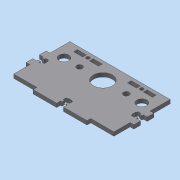
# Autodesk Inventor part: X-Anchor_Front-Outer
Saved by Autodesk Inventor 2016 SP1 (Build 200210100, 210)
## iProperties
Created: 2015-12-01
Part Number: X-Anchor_Front-Outer
Material: Generic
Document SubType Name: Modeling
Designer: Mohamed A.
Density: 1 g/cm^3
Appearance: Default
Author: Mohamed A.
Autodesk Inventor part; units mm, degrees
ref_plane "YZ Plane" through (0, 0, 0) normal (1, 0, 0) x (0, 1, 0)
ref_plane "XZ Plane" through (0, 0, 0) normal (0, 1, 0) x (-1, 0, 0)
ref_plane "XY Plane" through (0, 0, 0) normal (0, 0, 1) x (1, 0, 0)
sketch "Sketch1" plane through (0, 0, 0) normal (0, 0, 1) x (1, 0, 0)
  circle A0 centre (0, 5) radius 7.5
  line L0 (42.7333, 18.5) -> (-42.7333, 18.5)
  line L1 (-42.7333, -29) -> (42.7333, -29)
  circle A1 centre (18.5, 5) radius 2.25
  circle A2 centre (-18.5, 5) radius 2.25
  circle A3 centre (30.8333, 5) radius 3.9
  circle A4 centre (-30.8333, 5) radius 3.9
  line L2 (42.7333, 18.5) -> (42.7333, -29)
  line L3 (-42.7333, -29) -> (-42.7333, 18.5)
  circle A5 centre (0, 5) radius 13.5 construction
  line L4 (0, 41.7106) -> (0, -39.2634) construction
  dimension "d2" = 4.5
  dimension "d3" = 4.5
  dimension "d4" = 7.8
  dimension "d5" = 7.8
  dimension "d48" = 47.5
  dimension "d58" = 15
  dimension "d63" = 27
  dimension "d75" = 34
  dimension "d76" = 30.8333
  dimension "d77" = 85.4667
  dimension "d93" = 47.5
  dimension "d99" = 61.667
  constraints: 10 end point, 6 centre point, 3 vertical, 1 coincident, 1 perpendicular, 1 point on line, 6 other
  measures "d2" diameter of A1
  measures "d3" diameter of A2
  measures "d4" diameter of A3
  measures "d5" diameter of A4
  measures "d48" distance between parallel lines of L1 L0
  measures "d58" diameter of A0
  measures "d63" diameter of A5
  measures "d75" distance from line of A0.centre L1
  measures "d76" distance from line of A3.centre L4
  measures "d77" distance between parallel lines of L3 L2
  measures "d93" distance of L0.start L1.end
extrude "Extrusion1" add sketch "Sketch1" against normal blind 3
sketch "Sketch4" plane through (0, 0, 0) normal (0, 0, 1) x (1, 0, 0)
  line L0 (42.7333, 18.5) -> (39.7333, 18.5)
  line L1 (-42.7333, 18.5) -> (-39.7333, 18.5)
  line L2 (42.7333, -29) -> (21.3667, -29)
  line L3 (21.3667, -26) -> (39.7333, -26)
  line L4 (-42.7333, -29) -> (-21.3667, -29)
  line L5 (-21.3667, -29) -> (-21.3667, -26)
  line L6 (-21.3667, -26) -> (-39.7333, -26)
  line L7 (-42.7333, -23) -> (-42.7333, -29)
  line L8 (42.7333, 18.5) -> (39.7333, 18.5)
  line L9 (39.7333, 18.5) -> (39.7333, 2.6667)
  line L10 (39.7333, 2.6667) -> (42.7333, 2.6667)
  line L11 (42.7333, 2.6667) -> (42.7333, 18.5)
  line L12 (39.7333, -26) -> (39.7333, -13.1667)
  line L13 (39.7333, -13.1667) -> (42.7333, -13.1667)
  line L14 (-42.7333, 2.6667) -> (-39.7333, 2.6667)
  line L15 (-39.7333, 2.6667) -> (-39.7333, 18.5)
  line L16 (-39.7333, 18.5) -> (-42.7333, 18.5)
  line L17 (-42.7333, 18.5) -> (-42.7333, 2.6667)
  line L18 (-42.7333, -29) -> (-39.7333, -29)
  line L19 (-39.7333, -26) -> (-39.7333, -13.1667)
  line L20 (-39.7333, -13.1667) -> (-42.7333, -13.1667)
  line L21 (-42.7333, -13.1667) -> (-42.7333, -29)
  line L22 (21.3667, -29) -> (21.3667, -26)
  line L23 (-21.3667, -23) -> (-21.3667, -29)
  line L24 (-42.7333, 18.5) -> (-39.7333, 18.5)
  line L25 (-42.7333, -29) -> (42.7333, -29) projected
  line L26 (42.7333, 18.5) -> (-42.7333, 18.5) projected
  line L27 (50.1623, -5.25) -> (-50.4474, -5.25) construction
  line L28 (42.7333, -29) -> (42.7333, 18.5) projected
  line L29 (42.7333, -3.75) -> (34.7333, -3.75)
  line L30 (34.7333, -3.75) -> (34.7333, -6.75)
  line L31 (34.7333, -6.75) -> (42.7333, -6.75)
  line L32 (42.7333, -6.75) -> (42.7333, -3.75)
  circle A0 centre (0, 5) radius 13.5 construction
  circle A1 centre (0, 5) radius 7.5
  line L33 (42.7333, -2.6) -> (39.7333, -2.6)
  line L34 (39.7333, -2.6) -> (39.7333, -7.9)
  line L35 (39.7333, -7.9) -> (42.7333, -7.9)
  line L36 (42.7333, -7.9) -> (42.7333, -2.6)
  line L37 (35.3333, -2.6) -> (37.7333, -2.6)
  line L38 (37.7333, -2.6) -> (37.7333, -7.9)
  line L39 (37.7333, -7.9) -> (35.3333, -7.9)
  line L40 (35.3333, -7.9) -> (35.3333, -2.6)
  line L41 (0, 33.7344) -> (0, -36.9537) construction
  line L42 (-42.7333, 18.5) -> (-42.7333, -29) projected
  line L43 (-42.7333, -3.75) -> (-34.7333, -3.75)
  line L44 (-34.7333, -3.75) -> (-34.7333, -6.75)
  line L45 (-34.7333, -6.75) -> (-42.7333, -6.75)
  line L46 (-42.7333, -6.75) -> (-42.7333, -3.75)
  line L47 (-42.7333, -2.6) -> (-39.7333, -2.6)
  line L48 (-39.7333, -2.6) -> (-39.7333, -7.9)
  line L49 (-39.7333, -7.9) -> (-42.7333, -7.9)
  line L50 (-42.7333, -7.9) -> (-42.7333, -2.6)
  line L51 (-35.3333, -2.6) -> (-37.7333, -2.6)
  line L52 (-37.7333, -2.6) -> (-37.7333, -7.9)
  line L53 (-37.7333, -7.9) -> (-35.3333, -7.9)
  line L54 (-35.3333, -7.9) -> (-35.3333, -2.6)
  line L55 (42.7333, -29) -> (-42.7333, -29) projected
  line L56 (-1.5, -29) -> (1.5, -29)
  line L57 (1.5, -29) -> (1.5, -21)
  line L58 (1.5, -21) -> (-1.5, -21)
  line L59 (-1.5, -21) -> (-1.5, -29)
  line L60 (-2.65, -29) -> (2.65, -29)
  line L61 (2.65, -29) -> (2.65, -26)
  line L62 (2.65, -26) -> (-2.65, -26)
  line L63 (-2.65, -26) -> (-2.65, -29)
  line L64 (-2.65, -21.6) -> (2.65, -21.6)
  line L65 (2.65, -21.6) -> (2.65, -24)
  line L66 (2.65, -24) -> (-2.65, -24)
  line L67 (-2.65, -24) -> (-2.65, -21.6)
  line L68 (31.3, 16) -> (24.0167, 16) construction
  line L69 (11.4333, 16) -> (11.4333, 13) construction
  line L70 (11.4333, 13) -> (18.7167, 13) construction
  line L71 (31.3, 13) -> (31.3, 16) construction
  circle A2 centre (30.8333, 5) radius 3.9 projected
  line L72 (21.3667, 17.602) -> (21.3667, 7.8585) construction
  line L73 (18.7167, 16) -> (24.0167, 16) construction
  line L74 (24.0167, 16) -> (24.0167, 13) construction
  line L75 (24.0167, 13) -> (18.7167, 13) construction
  line L76 (18.7167, 13) -> (18.7167, 16) construction
  line L77 (18.7167, 16) -> (11.4333, 16) construction
  line L78 (24.0167, 13) -> (31.3, 13) construction
  circle A3 centre (21.3667, 14.5) radius 1.4
  line L79 (-31.3, 16) -> (-24.0167, 16) construction
  line L80 (-11.4333, 16) -> (-11.4333, 13) construction
  line L81 (-11.4333, 13) -> (-18.7167, 13) construction
  line L82 (-31.3, 13) -> (-31.3, 16) construction
  line L83 (-24.0167, 16) -> (-24.0167, 13) construction
  line L84 (-18.7167, 13) -> (-18.7167, 16) construction
  line L85 (-18.7167, 16) -> (-11.4333, 16) construction
  line L86 (-24.0167, 13) -> (-31.3, 13) construction
  circle A4 centre (-21.3667, 14.5) radius 1.4
  line L87 (42.7333, 18.5) -> (42.7333, -29) projected
  line L88 (42.7333, -13.1667) -> (42.7333, -29)
  line L89 (11.4247, 13) -> (11.4247, 16)
  line L90 (11.4247, 16) -> (18.7077, 16)
  line L91 (18.7077, 16) -> (18.7077, 13)
  line L92 (18.7077, 13) -> (11.4247, 13)
  line L93 (31.2907, 16) -> (31.2907, 13)
  line L94 (31.2907, 13) -> (24.0077, 13)
  line L95 (24.0077, 13) -> (24.0077, 16)
  line L96 (24.0077, 16) -> (31.2907, 16)
  line L97 (-18.7073, 13) -> (-18.7073, 16)
  line L98 (-18.7073, 16) -> (-11.4243, 16)
  line L99 (-11.4243, 16) -> (-11.4243, 13)
  line L100 (-11.4243, 13) -> (-18.7073, 13)
  line L101 (-24.0073, 16) -> (-24.0073, 13)
  line L102 (-24.0073, 13) -> (-31.2903, 13)
  line L103 (-31.2903, 13) -> (-31.2903, 16)
  line L104 (-31.2903, 16) -> (-24.0073, 16)
  dimension "d25" = 3
  dimension "d26" = 3
  dimension "d33" = 15.8333
  dimension "d59" = 8
  dimension "d60" = 3
  dimension "d61" = 47.5
  dimension "d62" = 27
  dimension "d65" = 5.3
  dimension "d66" = 2.4
  dimension "d68" = 5
  dimension "d69" = 3
  dimension "d70" = 8
  dimension "d71" = 5.3
  dimension "d74" = 5
  dimension "d78" = 3
  dimension "d81" = 3
  dimension "d82" = 11
  dimension "d83" = 19.8667
  dimension "d85" = 79.4667
  dimension "d86" = 85.4667
  dimension "d87" = 3
  dimension "d88" = 5.3
  dimension "d89" = 2.8
  dimension "d91" = 15.8333
  dimension "d92" = 21.3667
  dimension "d94" = 2.4
  dimension "d95" = 2.4
  dimension "d96" = 11.4333
  dimension "d97" = 7.2833
  dimension "d98" = 2.65
  constraints: 198 end point, 29 parallel, 25 horizontal, 21 symmetric about line, 15 collinear, 13 perpendicular, 10 point on line, 10 vertical, 4 centre point, 3 equal length, 1 concentric, 27 other
  measures "d25" distance of L2.end L3.start
  measures "d26" distance of L5.end L4.end
  measures "d33" distance from line of L0.start L10
  measures "d59" distance of L31.end L30.end
  measures "d60" distance of L30.end L29.end
  measures "d61" distance between parallel lines of L25 L26
  measures "d62" diameter of A0
  measures "d65" distance of L34.end L33.end
  measures "d66" distance of L38.end L39.end
  measures "d68" distance between parallel lines of L36 L38
  measures "d69" distance of L58.end L57.end
  measures "d70" distance of L57.end L56.end
  measures "d71" distance of L62.end L61.end
  measures "d74" distance between parallel lines of L60 L66
  measures "d78" distance between parallel lines of L17 L15
  measures "d81" distance of L69.end L69.start
  measures "d82" distance from line of L68 A2.centre
  measures "d83" distance between parallel lines of L69 L71
  measures "d85" distance between parallel lines of L15 L9
  measures "d86" distance between parallel lines of L42 L28
  measures "d87" distance between parallel lines of L9 L28
  measures "d88" distance of L74.end L70.end
  measures "d89" diameter of A3
  measures "d91" distance between parallel lines of L25 L13
  measures "d92" distance between parallel lines of L28 L22
  measures "d94" distance between parallel lines of L40 L38
  measures "d95" distance between parallel lines of L66 L64
  measures "d96" distance between parallel lines of L11 L71
  measures "d97" distance between parallel lines of L71 L74
  measures "d98" distance between parallel lines of L74 L72
extrude "Extrusion2" cut sketch "Sketch4" against normal through all contours L11 L10 L9 L0 | L15 L14 L17 L1 | L28 L29 L34 L33 | L28 L31 L34 L29 | L28 L35 L34 L31 | L34 L31 L38 L29 | L47 L48 L43 L42 | L38 L31 L40 L29 | L29 L40 L37 L38 | L43 L48 L45 L42 | L28 L2 L22 L3 L12 L13 | L38 L39 L40 L31 | L40 L31 L30 L29 | L45 L48 L49 L42 | L43 L52 L45 L48 | L52 L51 L54 L43 | L43 L54 L45 L52 | L20 L19 L6 L5 L4 L7 L21 | L45 L54 L53 L52 | L43 L44 L45 L54 | L25 L57 L62 L61 | L25 L59 L62 L57 | L25 L63 L62 L59 | L62 L59 L66 L57 | L66 L59 L64 L57 | L57 L64 L65 L66 | L66 L67 L64 L59 | L64 L59 L58 L57 | A1 | A3 | A4 | L89 L90 L91 L92 | L93 L94 L95 L96 | L97 L98 L99 L100 | L101 L102 L103 L104
equation "\"d48\" = d75 + 0.5 * d63"
equation "\"d33\" = 0.333333 * d61"
body "Solid1"
